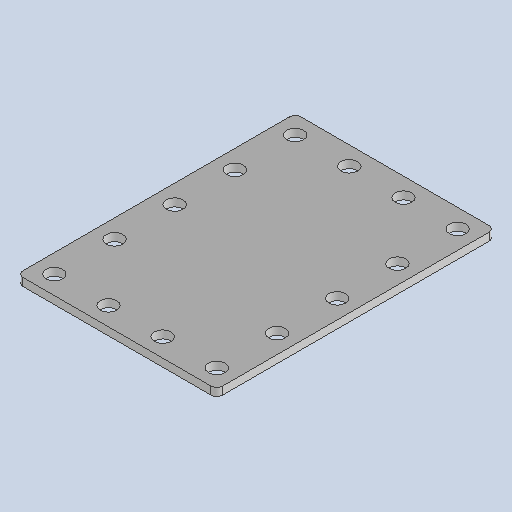
# Autodesk Inventor part: PRS 9607 charging flange rect_D1200 940
Saved by Autodesk Inventor 2026.2 (Build 302298000, 298)
## iProperties
Created: 2025-02-13
Part Number: PRS 9607 charging flange rect_D1200 940
Material: Steel
Document SubType Name: Sheet Metal
Designer: admin
Mass: 3436.88 g
Surface Area: 1231.62 cm^2
Volume: 437.819 cm^3
Density: 7.85 g/cm^3
Flat Pattern Width: 28.4 cm
Flat Pattern Length: 20.4 cm
Flat Pattern Area: 579.36 cm^2
Sheet Metal Rule: AISI304 4mm Die 32
Sheet Metal Width: 284,000 mm
Sheet Metal Length: 204,000 mm
Sheet Metal Area: 57936,000 mm^2
Appearance: Default
Author: pokla
Autodesk Inventor part; units mm, degrees
ref_plane "YZ Plane" through (0, 0, 0) normal (1, 0, 0) x (0, 1, 0)
ref_plane "XZ Plane" through (0, 0, 0) normal (0, 1, 0) x (-1, 0, 0)
ref_plane "XY Plane" through (0, 0, 0) normal (0, 0, 1) x (1, 0, 0)
sketch "Sketch2" plane through (0, 0, 0) normal (0, 0, 1) x (1, 0, 0)
  line L0 (-52, -92) -> (52, -92)
  line L1 (52, -92) -> (52, 92)
  line L2 (52, 92) -> (-52, 92)
  line L3 (-52, 92) -> (-52, -92)
  line L4 (-52, -92) -> (52, 92) construction
  line L5 (52, -92) -> (-52, 92) construction
  line L6 (-102, -142) -> (102, -142)
  line L7 (102, -142) -> (102, 142)
  line L8 (102, 142) -> (-102, 142)
  line L9 (-102, 142) -> (-102, -142)
  point P0 (0, 0)
  dimension "d31" = 50
  dimension "d60" = 184
  dimension "d61" = 104
  measures "d31" distance between parallel lines of L3 L9
  measures "d60" distance of L2.end L0.start
  measures "d61" distance of L0.start L0.end
extrude "Plate2" add sketch "Sketch2" along normal blind 8 contours L3 L2 L1 L0 | L9 L8 L7 L6
sketch "Sketch5" plane through (0, 0, 8) normal (0, 0, 1) x (1, 0, 0)
  line L0 (102, -142) -> (-102, -142) construction
  line L1 (102, 142) -> (102, -142) construction
  line L2 (-102, 142) -> (102, 142) construction
  line L3 (-102, -142) -> (-102, 142) construction
  line L4 (-83, 123) -> (83, 123) construction
  line L5 (83, 123) -> (83, -123) construction
  line L6 (83, -123) -> (-83, -123) construction
  line L7 (-83, -123) -> (-83, 123) construction
  line L8 (-27.6667, -123) -> (27.6667, -123)
  line L9 (27.6667, -123) -> (27.6667, 123) construction
  line L10 (27.6667, 123) -> (-27.6667, 123)
  line L11 (-27.6667, 123) -> (-27.6667, -123) construction
  line L12 (-27.6667, 0) -> (27.6667, 0) construction
  point P0 (0, 0)
  point P1 (0, -123)
  point P2 (-83, -61.5)
  point P3 (-83, 0)
  point P4 (-83, 61.5)
  point P5 (83, 61.5)
  point P6 (83, 0)
  point P7 (83, -61.5)
  point P8 (0, 0)
  dimension "d34" = 19
  dimension "d47" = 61.5
  dimension "d48" = 61.5
  dimension "d49" = 55.3333
  dimension "d50" = 55.3333
  constraints: 18 end point, 8 point on line, 6 midpoint, 5 coincident, 2 parallel, 2 symmetric about line, 1 horizontal, 1 horizontal alignment, 1 perpendicular, 3 other
  measures "d34" distance between parallel lines of L0 L6
  measures "d47" distance of point (-83, -61.5) point (-83, -123)
  measures "d48" distance of point (-83, 0) point (-83, -61.5)
  measures "d49" distance of L8.start point (-83, -123)
  measures "d50" distance of L8.end L8.start
fillet "Corner Round1" radius 6 4 edges at (-102, -142, 4) (-102, 142, 4) (102, 142, 4) (102, -142, 4)
hole "Hole1" at (-83, -123, 8) at (-83, -61.5, 8) at (-83, 0, 8) at (-83, 61.5, 8) at (-83, 123, 8) at (83, 123, 8) at (83, 61.5, 8) at (83, 0, 8) at (83, -61.5, 8) at (83, -123, 8) at (-27.6667, -123, 8) at (27.6667, 123, 8) at (27.6667, -123, 8) at (-27.6667, 123, 8) direction (0, 0, -1) diameter 17 end through all
equation "\"d47\" = d48"
equation "\"d49\" = d50"
equation "\"d60\" = ChargingHatch_width - 2 * Thickness"
equation "\"d61\" = ChargingHatch_hight - 2 * Thickness"
equation "\"d56\" = Thickness"
equation "\"d14\" = Thickness"
equation "\"BendReliefWidth\" = Thickness"
equation "\"BendReliefDepth\" = 0.5 * Thickness"
equation "\"CornerReliefSize\" = 4 * Thickness"
equation "\"MinimumRemnant\" = 2 * Thickness"
equation "\"TransitionRadius\" = BendRadius"
equation "\"JacobiRadiusSize\" = BendRadius"
equation "\"GapSize\" = Thickness"
equation "\"ChargingHatch_width\" = 200"
equation "\"Thickness\" = 8"
equation "\"ChargingHatch_hight\" = 120"
equation "\"BendRadius\" = 6"
body "Solid3"
